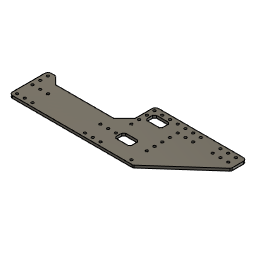
Parametric_z_plates_v9 (Autodesk Fusion 360 design; units mm, degrees)
Autodesk Fusion 360 part; units mm, degrees
note: some values were not read from the file. Set by a fixed rule: which sketch regions a step uses.
sketch "Sketch1" plane through (0, 0, 0) normal (0, 1, 0) x (1, 0, 0)
  line L0 (0, 0) -> (155, 0)
  line L1 (0, 0) -> (-100, 0)
  line L2 (0, 0) -> (0, 80)
  line L3 (0, 80) -> (-100, 80)
  line L4 (-100, 80) -> (-100, 0)
  line L5 (-100, 0) -> (-165, 0)
  line L6 (-165, 0) -> (-165, 80)
  line L7 (-125, 80) -> (-100, 80)
  line L8 (0, 80) -> (155, 80)
  line L9 (155, 80) -> (155, 0)
  line L10 (155, 80) -> (53, 80)
  line L11 (53, 80) -> (53, 160)
  line L12 (53, 160) -> (289.5, 160)
  line L13 (289.5, 160) -> (289.5, 120)
  line L14 (155, 80) -> (53, 80)
  line L15 (289.5, 120) -> (155, 120)
  line L16 (155, 120) -> (155, 80)
  line L17 (289.5, 120) -> (155, 0)
  line L18 (-165, 0) -> (-165, 100)
  line L19 (-165, 100) -> (-145, 100)
  line L20 (-145, 100) -> (-125, 80)
  line L21 (50.8, 80) -> (0, 80)
  line L22 (25.4, 80) -> (53, 107.6)
  dimension "d4" = 155
  dimension "d5" = 100
  dimension "d6" = 65
  dimension "d7" = 102
  dimension "d8" = 236.5
  dimension "d11" = 40
  dimension "d13" = 40
  dimension "d14" = 20
  dimension "d15" = 80
  dimension "d16" = 45
  constraint coincident L0.start L1.start
  constraint horizontal L0
  constraint parallel L0 L1
  constraint perpendicular L0 L2
  constraint perpendicular L2 L3
  constraint perpendicular L1 L4
  constraint perpendicular L4 L5
  constraint perpendicular L1 L6
  constraint perpendicular L4 L7
  constraint perpendicular L4 L8
  constraint perpendicular L8 L9
  constraint coincident L8 L10.end
  constraint perpendicular L10 L11
  constraint perpendicular L9 L12
  constraint perpendicular L12 L13
  constraint perpendicular L13 L14
  constraint perpendicular L9 L15
  constraint perpendicular L15 L16
  constraint perpendicular L15 L18
  constraint perpendicular L18 L19
  constraint coincident L8 L21.start
  constraint perpendicular L2 L21
  constraint midpoint L21 L22.start
  constraint coincident L11 L22.end
  measures "d4" distance of L0.start L0.end
  measures "d5" distance of L0.start L1.end
  measures "d6" distance of L1.end L5.end
  measures "d7" distance of L8.end L10.end
  measures "d8" distance of L11.end L12.end
  measures "d11" distance of L12.end L13.end
  measures "d13" distance of L18 L7.start
  measures "d14" distance of L18.end L19.end
  measures "d15" distance of L10.end L11.end
  measures "d16" angle of L21 L22
extrude "Extrude1" add sketch "Sketch1" along normal blind 6.3
fillet "Fillet1" radius 8.5 2 edges at (289.5, 3.15, -160) (53, 3.15, -160)
fillet "Fillet2" radius 8 2 edges at (-165, 3.15, 0) (-165, 3.15, -100)
sketch "Sketch2" plane through (0, 6.3, 0) normal (0, 1, 0) x (-1, 0, 0)
  arc A0 (157, -100) -> (165, -92) centre (157, -92) ccw
  line L0 (165, -92) -> (165, -8)
  arc A1 (165, -8) -> (157, 0) centre (157, -8) ccw
  line L1 (157, 0) -> (-155, 0)
  line L2 (-155, 0) -> (-289.5, -120)
  line L3 (-289.5, -120) -> (-289.5, -151.5)
  arc A2 (-289.5, -151.5) -> (-281, -160) centre (-281, -151.5) ccw
  line L4 (-281, -160) -> (-61.5, -160)
  arc A3 (-61.5, -160) -> (-53, -151.5) centre (-61.5, -151.5) ccw
  line L5 (-53, -151.5) -> (-53, -107.6)
  line L6 (-53, -107.6) -> (-25.4, -80)
  line L7 (-25.4, -80) -> (125, -80)
  line L8 (125, -80) -> (145, -100)
  line L9 (145, -100) -> (157, -100)
  circle A4 centre (155, -10) radius 3.1
  circle A5 centre (135, -10) radius 3.1
  circle A6 centre (115, -10) radius 3.1
  circle A7 centre (155, -50) radius 3.1
  circle A8 centre (135, -50) radius 3.1
  circle A9 centre (115, -50) radius 3.1
  circle A10 centre (155, -70) radius 3.1
  circle A11 centre (155, -90) radius 3.1
  line L10 (0, 0) -> (0, -80)
  circle A12 centre (-21, -10) radius 3.1
  line L11 (0, 0) -> (-155, 0)
  circle A13 centre (-41, -10) radius 3.1
  circle A14 centre (-61, -10) radius 3.1
  circle A15 centre (-21, -50) radius 3.1
  circle A16 centre (-41, -50) radius 3.1
  circle A17 centre (-61, -50) radius 3.1
  circle A18 centre (-61, -90) radius 3.1
  circle A19 centre (-61, -110) radius 3.1
  circle A20 centre (-61, -130) radius 3.1
  circle A21 centre (-61, -150) radius 3.1
  circle A22 centre (-81, -150) radius 3.1
  circle A23 centre (-101, -150) radius 3.1
  circle A24 centre (-121, -150) radius 3.1
  circle A25 centre (-141, -150) radius 3.1
  circle A26 centre (-141, -130) radius 3.1
  circle A27 centre (-141, -110) radius 3.1
  circle A28 centre (-141, -90) radius 3.1
  circle A29 centre (-141, -70) radius 3.1
  circle A30 centre (-141, -50) radius 3.1
  circle A31 centre (-161, -150) radius 3.1
  circle A32 centre (-161, -130) radius 3.1
  circle A33 centre (-181, -150) radius 3.1
  circle A34 centre (-181, -130) radius 3.1
  circle A35 centre (-271.5, -130) radius 3.1
  circle A36 centre (-271.5, -150) radius 3.1
  circle A37 centre (-251.5, -130) radius 3.1
  circle A38 centre (-251.5, -150) radius 3.1
  dimension "d21" = 6.2
  dimension "d22" = 10
  dimension "d23" = 10
  dimension "d26" = -40
  dimension "d27" = -40
  dimension "d30" = 0
  dimension "d31" = -40
  dimension "d32" = 6.2
  dimension "d33" = 10
  dimension "d34" = 21
  dimension "d37" = -40
  dimension "d38" = -40
  dimension "d41" = 0
  dimension "d42" = -40
  dimension "d45" = 0
  dimension "d46" = -60
  dimension "d49" = -60
  dimension "d50" = 0
  dimension "d53" = -20
  dimension "d54" = 0
  dimension "d57" = 0
  dimension "d58" = 100
  dimension "d61" = -40
  dimension "d62" = 0
  dimension "d72" = 18
  dimension "d73" = 18
  dimension "d74" = 20
  dimension "d75" = 20
  dimension "d111" = 6.2
  dimension "d112" = 6.2
  dimension "d113" = 6.2
  dimension "d114" = 6.2
  measures "d21" diameter of A4
  measures "d22" distance of L0 A4.centre
  measures "d23" distance of L1 A4.centre
  measures "d32" diameter of A12
  measures "d33" distance of A12.centre L11
  measures "d34" distance of L10 A12.centre
  measures "d72" distance of L3 A36.centre
  measures "d73" distance of L3 A35.centre
  measures "d74" distance of A35.centre A37.centre
  measures "d75" distance of A36.centre A38.centre
  measures "d111" diameter of A37
  measures "d112" diameter of A38
  measures "d113" diameter of A36
  measures "d114" diameter of A35
extrude "Extrude2" cut sketch "Sketch2" against normal through all contours A4 | A5 | A6 | A7 | A8 | A9 | A10 | A11 | A12 | A13 | A14 | A15 | A16 | A17 | A18 | A19 | A20 | A21 | A22 | A23 | A24 | A25 | A26 | A27 | A28 | A29 | A30 | A31 | A32 | A33 | A34 | A35 | A36 | A37 | A38
sketch "Sketch3" plane through (0, 6.3, 0) normal (0, 1, 0) x (-1, 0, 0)
  circle A0 centre (155, -50) radius 3.1
  circle A1 centre (135, -10) radius 3.1
  circle A2 centre (-21, -10) radius 3.1
  circle A3 centre (-61, -90) radius 3.1
  circle A4 centre (-81, -150) radius 3.1
  circle A5 centre (-141, -70) radius 3.1
  circle A6 centre (-141, -150) radius 3.1
  circle A7 centre (-181, -150) radius 3.1
  circle A8 centre (-271.5, -150) radius 3.1
  circle A9 centre (-251.5, -130) radius 3.1
  circle A10 centre (-161, -150) radius 3.1
  circle A11 centre (-141, -90) radius 3.1
  circle A12 centre (-101, -150) radius 3.1
  circle A13 centre (-61, -110) radius 3.1
  circle A14 centre (-41, -10) radius 3.1
  circle A15 centre (155, -10) radius 3.1
  circle A16 centre (115, -50) radius 3.1
  circle A17 centre (155, -70) radius 3.1
  circle A18 centre (115, -10) radius 3.1
  circle A19 centre (-21, -50) radius 3.1
  circle A20 centre (-61, -50) radius 3.1
  circle A21 centre (-61, -150) radius 3.1
  circle A22 centre (-141, -50) radius 3.1
  circle A23 centre (-141, -130) radius 3.1
  circle A24 centre (-181, -130) radius 3.1
  circle A25 centre (-271.5, -130) radius 3.1
  circle A26 centre (-251.5, -150) radius 3.1
  circle A27 centre (-161, -130) radius 3.1
  circle A28 centre (-141, -110) radius 3.1
  circle A29 centre (-121, -150) radius 3.1
  circle A30 centre (-61, -130) radius 3.1
  circle A31 centre (-61, -10) radius 3.1
  circle A32 centre (-41, -50) radius 3.1
  circle A33 centre (135, -50) radius 3.1
  circle A34 centre (155, -90) radius 3.1
  arc A35 (157, -100) -> (165, -92) centre (157, -92) ccw
  line L0 (165, -92) -> (165, -8)
  arc A36 (165, -8) -> (157, 0) centre (157, -8) ccw
  line L1 (157, 0) -> (-155, 0)
  line L2 (-155, 0) -> (-289.5, -120)
  line L3 (-289.5, -120) -> (-289.5, -151.5)
  arc A37 (-289.5, -151.5) -> (-281, -160) centre (-281, -151.5) ccw
  line L4 (-281, -160) -> (-61.5, -160)
  arc A38 (-61.5, -160) -> (-53, -151.5) centre (-61.5, -151.5) ccw
  line L5 (-53, -151.5) -> (-53, -107.6)
  line L6 (-53, -107.6) -> (-25.4, -80)
  line L7 (-25.4, -80) -> (125, -80)
  line L8 (125, -80) -> (145, -100)
  line L9 (145, -100) -> (157, -100)
  circle A39 centre (-271.5, -130.0092) radius 3.1
  circle A40 centre (-271.5, -150.0092) radius 3.1
  circle A41 centre (-231.5, -130) radius 3.1
  circle A42 centre (-231.5, -150) radius 3.1
  dimension "d76" = 6.2
  dimension "d77" = 6.2
  dimension "d78" = 20
  dimension "d79" = 20
  dimension "d106" = 20
  dimension "d107" = 0
  measures "d76" diameter of A39
  measures "d77" diameter of A40
  measures "d78" distance of A9.centre A39.centre
  measures "d79" distance of A26.centre A40.centre
extrude "Extrude3" cut sketch "Sketch3" against normal through all contours A8 A40 | A25 A39
sketch "Sketch4" plane through (0, 6.3, 0) normal (0, 1, 0) x (-1, 0, 0)
  circle A0 centre (155, -50) radius 3.1
  circle A1 centre (135, -10) radius 3.1
  circle A2 centre (-21, -10) radius 3.1
  circle A3 centre (-61, -90) radius 3.1
  circle A4 centre (-81, -150) radius 3.1
  circle A5 centre (-141, -70) radius 3.1
  circle A6 centre (-141, -150) radius 3.1
  circle A7 centre (-181, -150) radius 3.1
  circle A8 centre (-251.5, -130) radius 3.1
  circle A9 centre (-161, -150) radius 3.1
  circle A10 centre (-141, -90) radius 3.1
  circle A11 centre (-101, -150) radius 3.1
  circle A12 centre (-61, -110) radius 3.1
  circle A13 centre (-41, -10) radius 3.1
  circle A14 centre (155, -10) radius 3.1
  circle A15 centre (115, -50) radius 3.1
  circle A16 centre (155, -70) radius 3.1
  circle A17 centre (115, -10) radius 3.1
  circle A18 centre (-21, -50) radius 3.1
  circle A19 centre (-61, -50) radius 3.1
  circle A20 centre (-61, -150) radius 3.1
  circle A21 centre (-141, -50) radius 3.1
  circle A22 centre (-141, -130) radius 3.1
  circle A23 centre (-181, -130) radius 3.1
  circle A24 centre (-251.5, -150) radius 3.1
  circle A25 centre (-161, -130) radius 3.1
  circle A26 centre (-141, -110) radius 3.1
  circle A27 centre (-121, -150) radius 3.1
  circle A28 centre (-61, -130) radius 3.1
  circle A29 centre (-61, -10) radius 3.1
  circle A30 centre (-41, -50) radius 3.1
  circle A31 centre (135, -50) radius 3.1
  circle A32 centre (155, -90) radius 3.1
  arc A33 (157, -100) -> (165, -92) centre (157, -92) ccw
  line L0 (165, -92) -> (165, -8)
  arc A34 (165, -8) -> (157, 0) centre (157, -8) ccw
  line L1 (157, 0) -> (-155, 0)
  line L2 (-155, 0) -> (-289.5, -120)
  line L3 (-289.5, -120) -> (-289.5, -151.5)
  arc A35 (-289.5, -151.5) -> (-281, -160) centre (-281, -151.5) ccw
  line L4 (-281, -160) -> (-61.5, -160)
  arc A36 (-61.5, -160) -> (-53, -151.5) centre (-61.5, -151.5) ccw
  line L5 (-53, -151.5) -> (-53, -107.6)
  line L6 (-53, -107.6) -> (-25.4, -80)
  line L7 (-25.4, -80) -> (125, -80)
  line L8 (125, -80) -> (145, -100)
  line L9 (145, -100) -> (157, -100)
  line L10 (-74, -142) -> (-105, -142)
  line L11 (-109, -138) -> (-109, -122)
  line L12 (-105, -118) -> (-73, -118)
  line L13 (-69, -122) -> (-69, -137)
  line L14 (-69, -142) -> (-109, -118) construction
  line L15 (-109, -142) -> (-69, -118) construction
  line L16 (-69, -137) -> (-74, -142)
  line L17 (-69, -122) -> (-73, -118)
  line L18 (-109, -122) -> (-105, -118)
  line L19 (-109, -138) -> (-105, -142)
  line L20 (-105, -38) -> (-73, -38)
  line L21 (-109, -42) -> (-105, -38)
  line L22 (-109, -58) -> (-109, -42)
  line L23 (-109, -58) -> (-105, -62)
  line L24 (-74, -62) -> (-105, -62)
  line L25 (-69, -62) -> (-109, -38) construction
  line L26 (-69, -57) -> (-74, -62)
  line L27 (-69, -42) -> (-69, -57)
  line L28 (-69, -42) -> (-73, -38)
  arc A37 (-274.6, -150.0053) -> (-268.4, -150.0039) centre (-271.5, -150.0092) ccw
  arc A38 (-268.4, -150.0039) -> (-274.6, -150.0053) centre (-271.5, -150) ccw
  arc A39 (-274.6, -130.0053) -> (-268.4, -130.0039) centre (-271.5, -130.0092) ccw
  arc A40 (-268.4, -130.0039) -> (-274.6, -130.0053) centre (-271.5, -130) ccw
  point P0 (-89, -130)
  dimension "d81" = 40
  dimension "d82" = 24
  dimension "d83" = 16
  dimension "d84" = 18
  dimension "d85" = 5
  dimension "d86" = 5
  dimension "d87" = 4
  dimension "d88" = 4
  dimension "d89" = 4
  dimension "d90" = 4
  dimension "d91" = 4
  dimension "d92" = 4
  dimension "d95" = 0
  dimension "d96" = 80
  constraint horizontal L10
  constraint perpendicular L10 L11
  constraint parallel L10 L12
  constraint parallel L11 L13
  constraint coincident L14 P0
  constraint coincident L15 P0
  constraint coincident L14.start L13
  constraint coincident L14.start L10
  constraint coincident L15.end L13
  constraint coincident L15.end L12
  constraint coincident L14.end L11
  constraint coincident L14.end L12
  constraint coincident L15.start L11
  constraint coincident L15.start L10
  measures "d81" distance of L14.end L15.end
  measures "d82" distance of L15.start L14.end
  measures "d83" distance of L5 L13
  measures "d84" distance of L4 L10
  measures "d85" distance of L14.start L13.end
  measures "d86" distance of L14.start L10.start
  measures "d87" distance of L15.end L13.start
  measures "d88" distance of L15.end L12.end
  measures "d89" distance of L14.end L11.end
  measures "d90" distance of L14.end L12.start
  measures "d91" distance of L15.start L11.start
  measures "d92" distance of L15.start L10.end
extrude "Extrude4" cut sketch "Sketch4" against normal through all contours L10 L11 L12 L13 L16 L17 L18 L19 | L20 L21 L22 L23 L24 L26 L27 L28
fillet "Fillet3" radius 5 1 edges at (289.5, 3.15, -120)
fillet "Fillet4" radius 5 1 edges at (-145, 3.15, -100)
sketch "Sketch5" plane through (0, 6.3, 0) normal (0, 1, 0) x (-1, 0, 0)
  arc A0 (143.5355, -98.5355) -> (147.0711, -100) centre (147.0711, -95) ccw
  line L0 (147.0711, -100) -> (157, -100)
  arc A1 (157, -100) -> (165, -92) centre (157, -92) ccw
  line L1 (165, -92) -> (165, -8)
  arc A2 (165, -8) -> (157, 0) centre (157, -8) ccw
  line L2 (157, 0) -> (-155, 0)
  line L3 (-155, 0) -> (-287.8287, -118.5089)
  arc A3 (-287.8287, -118.5089) -> (-289.5, -122.2398) centre (-284.5, -122.2398) ccw
  line L4 (-289.5, -122.2398) -> (-289.5, -151.5)
  arc A4 (-289.5, -151.5) -> (-281, -160) centre (-281, -151.5) ccw
  line L5 (-281, -160) -> (-61.5, -160)
  arc A5 (-61.5, -160) -> (-53, -151.5) centre (-61.5, -151.5) ccw
  line L6 (-53, -151.5) -> (-53, -107.6)
  line L7 (-53, -107.6) -> (-25.4, -80)
  line L8 (-25.4, -80) -> (125, -80)
  line L9 (125, -80) -> (143.5355, -98.5355)
  line L10 (-73, -118) -> (-69, -122)
  line L11 (-69, -122) -> (-69, -137)
  line L12 (-69, -137) -> (-74, -142)
  line L13 (-74, -142) -> (-105, -142)
  line L14 (-105, -142) -> (-109, -138)
  line L15 (-109, -138) -> (-109, -122)
  line L16 (-109, -122) -> (-105, -118)
  line L17 (-105, -118) -> (-73, -118)
  line L18 (-105, -62) -> (-109, -58)
  line L19 (-109, -58) -> (-109, -42)
  line L20 (-109, -42) -> (-105, -38)
  line L21 (-105, -38) -> (-73, -38)
  line L22 (-73, -38) -> (-69, -42)
  line L23 (-69, -42) -> (-69, -57)
  line L24 (-69, -57) -> (-74, -62)
  line L25 (-74, -62) -> (-105, -62)
  circle A6 centre (155, -50) radius 3.1
  circle A7 centre (135, -10) radius 3.1
  circle A8 centre (-21, -10) radius 3.1
  circle A9 centre (-61, -90) radius 3.1
  circle A10 centre (-81, -150) radius 3.1
  circle A11 centre (-141, -70) radius 3.1
  circle A12 centre (-141, -150) radius 3.1
  circle A13 centre (-181, -150) radius 3.1
  circle A14 centre (-251.5, -130) radius 3.1
  circle A15 centre (-161, -150) radius 3.1
  circle A16 centre (-141, -90) radius 3.1
  circle A17 centre (-101, -150) radius 3.1
  circle A18 centre (-61, -110) radius 3.1
  circle A19 centre (-41, -10) radius 3.1
  circle A20 centre (155, -10) radius 3.1
  circle A21 centre (115, -50) radius 3.1
  circle A22 centre (155, -70) radius 3.1
  circle A23 centre (115, -10) radius 3.1
  circle A24 centre (-21, -50) radius 3.1
  circle A25 centre (-61, -50) radius 3.1
  circle A26 centre (-61, -150) radius 3.1
  circle A27 centre (-141, -50) radius 3.1
  circle A28 centre (-141, -130) radius 3.1
  circle A29 centre (-181, -130) radius 3.1
  circle A30 centre (-251.5, -150) radius 3.1
  circle A31 centre (-161, -130) radius 3.1
  circle A32 centre (-141, -110) radius 3.1
  circle A33 centre (-121, -150) radius 3.1
  circle A34 centre (-61, -130) radius 3.1
  circle A35 centre (-61, -10) radius 3.1
  circle A36 centre (-41, -50) radius 3.1
  circle A37 centre (135, -50) radius 3.1
  circle A38 centre (155, -90) radius 3.1
  line L26 (-61, -10) -> (-141, -10)
  line L27 (-141, -10) -> (-141, -50)
  circle A39 centre (-141, -10) radius 3.1
  arc A40 (-274.6, -130.0053) -> (-268.4, -130.0039) centre (-271.5, -130.0092) ccw
  arc A41 (-268.4, -130.0039) -> (-274.6, -130.0053) centre (-271.5, -130) ccw
  arc A42 (-274.6, -150.0053) -> (-268.4, -150.0039) centre (-271.5, -150.0092) ccw
  arc A43 (-268.4, -150.0039) -> (-274.6, -150.0053) centre (-271.5, -150) ccw
  dimension "d102" = 6.2
  constraint coincident A35.centre L26.start
  constraint parallel L2 L26
  constraint coincident A27.centre L27.end
  constraint perpendicular L26 L27
  constraint coincident L26.end L27.start
  measures "d102" diameter of A39
extrude "Extrude5" cut sketch "Sketch5" against normal through all contours L26 L27 A39 | L26 L27 A39
extrude "Extrude6" cut sketch "Sketch3" against normal through all contours A41 | A42
fillet "Fillet5" radius 5 1 edges at (155, 3.15, 0)
equation "Holes = 6.2 mm"
equation "Thickness = 6.3 mm"
equation "Hieight = 100 mm" comment "Z clearance"
equation "d5 = Hieight"
equation "d8 = Zrails"
equation "d9 = Thickness"
equation "Zrails = 236.5 mm" comment "Lenth of rails minus 13.5, Recommended not to go over 300mm"
equation "d21 = Holes"
equation "d32 = Holes"
equation "d76 = Holes"
equation "d77 = Holes"
equation "d86 = d85"
equation "d88 = d87"
equation "d90 = d89"
equation "d92 = d91"
equation "d102 = Holes"
equation "d111 = Holes"
equation "d112 = Holes"
equation "d113 = Holes"
equation "d114 = Holes"
